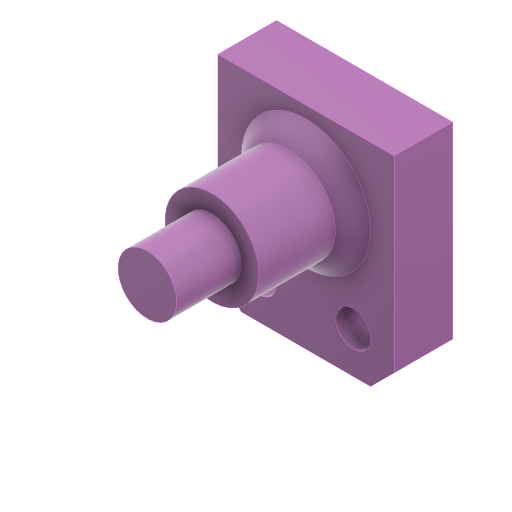
# Autodesk Inventor part: Концентратор
Saved by Autodesk Inventor 2023 (Build 270158000, 158)
## iProperties
Created: 2023-03-29
Part Number: Концентратор
Material: Типовые
Document SubType Name: Modeling
Designer: Admin
Density: 1 g/cm^3
Appearance: По умолчанию
Author: Admin
Autodesk Inventor part; units mm, degrees
ref_plane "YZ Plane" through (0, 0, 0) normal (1, 0, 0) x (0, 1, 0)
ref_plane "XZ Plane" through (0, 0, 0) normal (0, 1, 0) x (-1, 0, 0)
ref_plane "XY Plane" through (0, 0, 0) normal (0, 0, 1) x (1, 0, 0)
sketch "Эскиз1" plane through (0, 0, 0) normal (0, 0, 1) x (1, 0, 0)
  line L0 (7.5, -9.5) -> (5.5, -11.5)
  line L1 (5.5, -11.5) -> (-5.5, -11.5)
  circle A0 centre (4, -8) radius 1.5
  circle A1 centre (-4, -8) radius 1.5
  line L2 (-7.5, -9.5) -> (-5.5, -11.5)
  circle A2 centre (0, 0) radius 2.5
  line L3 (7.5, 6.5) -> (7.5, -9.5)
  line L4 (-7.5, 6.5) -> (7.5, -11.5) construction
  line L5 (-7.5, -11.5) -> (7.5, 6.5) construction
  line L6 (-7.5, -9.5) -> (-7.5, 6.5)
  circle A3 centre (0, 0) radius 8 construction
  line L7 (-7.5, 6.5) -> (7.5, 6.5)
  circle A4 centre (0, 0) radius 4
  point P0 (2.6268, 7.5565)
  point P1 (0, 6.5)
  dimension "d18" = 16
  dimension "d7" = 15
  dimension "d8" = 16
  dimension "d9" = 11
  dimension "d10" = 5
  dimension "d11" = 3
  dimension "d16" = 45
  dimension "d17" = 45
  dimension "d19" = 16
  dimension "d28" = 8
  dimension "d32" = 6.5
  dimension "d33" = 3.5
  dimension "d34" = 3.5
  dimension "d35" = 3.5
  dimension "d36" = 3.5
  constraints: 16 end point, 4 centre point, 4 point on line, 3 coincident, 2 horizontal, 2 vertical, 1 equal radius, 1 midpoint, 1 vertical alignment, 3 other
  measures "d7" distance of L4.start L3.start
  measures "d8" distance of L3.start L0.start
  measures "d9" distance of L1.start L1.end
  measures "d10" diameter of A2
  measures "d11" diameter of A0
  measures "d16" angle of L2 L6
  measures "d17" angle of L0 L3
  measures "d19" distance of L2.start L4.start
  measures "d28" diameter of A4
  measures "d32" distance from line of point (0, 0) L7
  measures "d33" distance from line of L1 point (4, -8)
  measures "d34" distance from line of L3 point (4, -8)
  measures "d35" distance from line of L1 A1.centre
  measures "d36" distance from line of L6 A1.centre
extrude "Выдавливание1" add sketch "Эскиз1" along normal blind 18.5 contours A2
extrude "Выдавливание2" add sketch "Эскиз1" along normal blind 5 contours L0 L1 L2 L6 L7 L3 | A2 | A4
extrude "Выдавливание3" add sketch "Эскиз1" along normal blind 13 contours A4
chamfer "Фаска1" distance 1.5 angle 45 1 edges at (-4, 0, 5)
